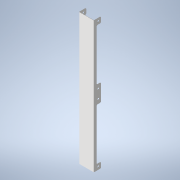
# Autodesk Inventor part: Yderskal - Sheet metal
Saved by Autodesk Inventor 2020 (Build 240168000, 168)
## iProperties
Created: 2021-05-19
Part Number: Yderskal - Sheet metal
Material: Generic
Document SubType Name: Sheet Metal
Designer: 6128059
Density: 1 g/cm^3
Sheet Metal Rule: Default_mm
Appearance: Default
Author: 6128059
Autodesk Inventor part; units mm, degrees
ref_plane "YZ Plane" through (0, 0, 0) normal (1, 0, 0) x (0, 1, 0)
ref_plane "XZ Plane" through (0, 0, 0) normal (0, 1, 0) x (-1, 0, 0)
sketch "Sketch1" plane through (0, 0, 0) normal (0, 0, 1) x (1, 0, 0)
  line L0 (25, -120) -> (25, 120)
  line L1 (0.1, 120) -> (24.9, 120) construction
  line L2 (0, 120) -> (0, -120)
  line L3 (24.9, -120) -> (0.1, -120) construction
  line L4 (25, 120) -> (0, 120) construction
  line L5 (0, 120) -> (0, 120) construction
  line L6 (0, -120) -> (25, -120) construction
  line L7 (25, -120) -> (25, -120) construction
  line L8 (25, 120) -> (0, 120)
  line L9 (25, -120) -> (0, -120)
  line L10 (25, 120) -> (25, 120) construction
  line L11 (0, 120) -> (0, -120)
  line L12 (25, -120) -> (25, 120)
  line L13 (0, -120) -> (0, -120) construction
  point P0 (0, 0)
  dimension "d17" = 0
  dimension "d18" = 0
  measures "d17" distance between parallel lines of L9 L3
  measures "d18" distance between parallel lines of L1 L8
extrude "Plate1" add sketch "Sketch1" along normal blind 0.5
sketch "Sketch2" plane through (25.5, -120, -0.5) normal (1, 0, 0) x (0, 1, 0)
  line L0 (240, 0) -> (0, 0)
  line L1 (0, 0) -> (0, -12)
  line L2 (0, -12) -> (240, -12)
  line L3 (240, -12) -> (240, 0)
  constraints: 6 end point, 1 horizontal, 1 perpendicular, 1 vertical
edge flange "Flange1" height 13 angle 90 thickness 0.5 bend radius 0.5 thickness toward (1, 0, 0) relief tear relief width 0.5 relief depth 0.25 corner gap 0.5 corner form 0 edges at (25, 0, 0) (0, 0, 0) wall of the first edge with corners at (25.5, 120, -0.5) (25.5, -120, -0.5) (25.5, -120, -12.5) (25.5, 120, -12.5)
bend "Bend1"
corner "Corner1"
sketch "Sketch3" plane through (26, -125, -12.5) normal (1, 0, 0) x (0, 0, -1)
  line L0 (-6, 10) -> (-6, 115) construction
  circle A0 centre (-6, 10) radius 2 construction
  circle A1 centre (-6, 115) radius 2 construction
  line L1 (-6, 135) -> (-6, 240) construction
  circle A2 centre (-6, 135) radius 2 construction
  circle A3 centre (-6, 240) radius 2 construction
  line L2 (0, 5) -> (-12, 5) projected
  line L3 (-12, 245) -> (0, 245) projected
  line L4 (0, 245) -> (0, 5) projected
  line L5 (0, 5) -> (0, 245) projected
  line L6 (0, 15) -> (-8, 15)
  line L7 (-8, 15) -> (-8, 107.5)
  line L8 (-8, 107.5) -> (0, 107.5)
  line L9 (0, 142.5) -> (-8, 142.5)
  line L10 (-8, 142.5) -> (-8, 235)
  line L11 (-8, 235) -> (0, 235)
  point P0 (-12.5, 125)
  point P1 (-6, 245)
  point P2 (-8, 61.25)
  point P3 (-8, 188.75)
  dimension "d11" = 4
  dimension "d12" = 4
  dimension "d13" = 105
  dimension "d14" = 105
  dimension "d19" = 5
  dimension "d20" = 5
  dimension "d21" = 10
  dimension "d22" = 7.5
  dimension "d23" = 7.5
  dimension "d24" = 10
  dimension "d25" = 8
  constraints: 16 end point, 6 point on line, 5 perpendicular, 4 centre point, 4 coincident, 3 midpoint, 3 vertical alignment, 2 equal radius, 2 vertical
  measures "d11" diameter of A0
  measures "d12" diameter of A1
  measures "d13" distance of L0.start L0.end
  measures "d14" distance of L1.start L1.end
  measures "d19" distance from line of L2 L0.start
  measures "d20" distance from line of L3 L1.end
  measures "d21" distance between parallel lines of L3 L11
  measures "d22" distance from line of A2.centre L9
  measures "d23" distance from line of L8 L0.end
  measures "d24" distance between parallel lines of L2 L6
  measures "d25" distance between parallel lines of L4 L7
extrude "Cut1" cut sketch "Sketch3" against normal blind 40
fillet "Fillet1" radius 2 20 edges at (25.75, -120, -12.5) (25.75, 110, -12.5) (25.75, 110, -4.5) (25.75, 17.5, -12.5) (25.75, 17.5, -4.5) (25.75, -17.5, -12.5) (25.75, -17.5, -4.5) (25.75, -110, -4.5) (25.75, -110, -12.5) (25.75, 120, -12.5) (-0.75, -17.5, -12.5) (-0.75, 120, -12.5) (-0.75, -110, -12.5) (-0.75, -110, -4.5) (-0.75, -17.5, -4.5) (-0.75, 17.5, -12.5) (-0.75, 17.5, -4.5) (-0.75, 110, -12.5) (-0.75, -120, -12.5) (-0.75, 110, -4.5)
sketch "Sketch4" plane through (26, -120, -0.5) normal (1, 0, 0) x (0, 0, -1)
  arc A0 (10, 230) -> (12, 232) centre (10, 232) ccw projected
  line L0 (10, 230) -> (6, 230) projected
  arc A1 (6, 230) -> (4, 228) centre (6, 228) ccw projected
  line L1 (4, 228) -> (4, 139.5) projected
  arc A2 (4, 139.5) -> (6, 137.5) centre (6, 139.5) ccw projected
  line L2 (6, 137.5) -> (10, 137.5) projected
  arc A3 (12, 135.5) -> (10, 137.5) centre (10, 135.5) ccw projected
  line L3 (12, 135.5) -> (12, 104.5) projected
  arc A4 (10, 102.5) -> (12, 104.5) centre (10, 104.5) ccw projected
  line L4 (10, 102.5) -> (6, 102.5) projected
  arc A5 (6, 102.5) -> (4, 100.5) centre (6, 100.5) ccw projected
  line L5 (4, 100.5) -> (4, 12) projected
  arc A6 (4, 12) -> (6, 10) centre (6, 12) ccw projected
  line L6 (6, 10) -> (10, 10) projected
  arc A7 (12, 8) -> (10, 10) centre (10, 8) ccw projected
  line L7 (12, 8) -> (12, 2) projected
  arc A8 (10, 0) -> (12, 2) centre (10, 2) ccw projected
  line L8 (10, 0) -> (0, 0) projected
  line L9 (0, 0) -> (0, 240) projected
  line L10 (0, 240) -> (10, 240) projected
  arc A9 (12, 238) -> (10, 240) centre (10, 238) ccw projected
  line L11 (12, 238) -> (12, 232) projected
  point P0 (-0.5, 120)
  point P1 (7, 7.25)
  point P2 (7, 112.25)
  point P3 (7, 127.75)
  point P4 (7, 232.75)
  dimension "d29" = 5
  dimension "d30" = 7.25
  dimension "d33" = 7.25
  dimension "d65" = 105
  dimension "d66" = 105
  constraints: 3 vertical alignment
  measures "d29" distance from line of L11 point (7, 232.75)
  measures "d30" distance from line of L10 point (7, 232.75)
  measures "d33" distance from line of L8 point (7, 7.25)
  measures "d65" distance of point (7, 7.25) point (7, 112.25)
  measures "d66" distance of point (7, 232.75) point (7, 127.75)
hole "Hole1" at (26, -112.75, -7.5) at (26, 112.75, -7.5) at (26, 7.75, -7.5) at (26, -7.75, -7.5) direction (-1, 0, 0) diameter 3.242 depth 11.8 thread size "M4x0.7" class "6H" standard "ISO Metric profile"
ref_plane "Work Plane1" through (12.5, -120, -12.5) normal (-1, 0, 0) x (0, 0, 1)
mirror "Mirror1" about plane through (12.5, -120, -12.5) normal (-1, 0, 0) of "Hole1"
equation "\"d12\" = d11"
equation "\"d20\" = d19"
equation "\"d23\" = d22"
equation "\"d24\" = d21"
equation "\"d0\" = Thickness"
equation "\"d1\" = BendReliefWidth"
equation "\"d2\" = BendReliefDepth"
equation "\"d3\" = MinimumRemnant"
equation "\"d4\" = TransitionRadius"
equation "\"d7\" = BendRadius"
equation "\"d8\" = CornerReliefSize"
equation "\"d9\" = GapSize"
equation "\"d10\" = JacobiRadiusSize"
equation "\"d33\" = d30"
equation "\"BendRadius\" = Thickness"
equation "\"BendReliefWidth\" = Thickness"
equation "\"BendReliefDepth\" = 0.5 * Thickness"
equation "\"CornerReliefSize\" = 4 * Thickness"
equation "\"MinimumRemnant\" = 2 * Thickness"
equation "\"TransitionRadius\" = BendRadius"
equation "\"JacobiRadiusSize\" = BendRadius"
equation "\"GapSize\" = Thickness"
equation "\"Thickness\" = 0.5"
body "Solid1"
